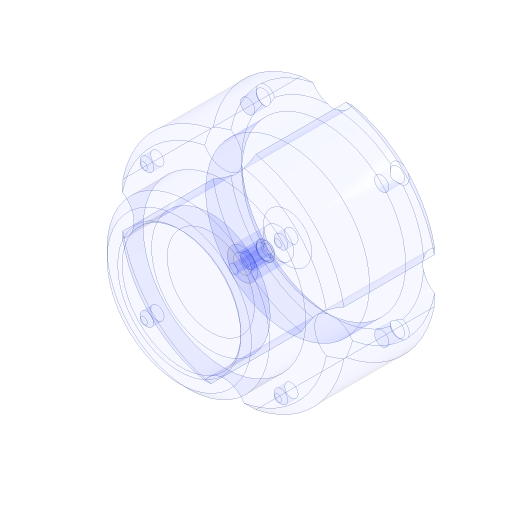
# Autodesk Inventor part: centrifugetool_3.2mm_funnel_v3
Saved by Autodesk Inventor 2024 (Build 280153000, 153)
## iProperties
Created: 2021-10-27
Part Number: centrifugetool_3.2mm_funnel_v3
Material: Generic
Document SubType Name: Modeling
Designer: to172
Density: 1 g/cm^3
Appearance: Clear - Blue
Author: to172
Autodesk Inventor part; units mm, degrees
ref_plane "YZ Plane" through (0, 0, 0) normal (1, 0, 0) x (0, 1, 0)
ref_plane "XZ Plane" through (0, 0, 0) normal (0, 1, 0) x (-1, 0, 0)
ref_plane "XY Plane" through (0, 0, 0) normal (0, 0, 1) x (1, 0, 0)
sketch "Sketch1" plane through (0, 0, 0) normal (0, 0, 1) x (1, 0, 0)
  circle A0 centre (0, 0) radius 12.5
  dimension "d0" = 25
  constraints: 1 centre point, 1 coincident
  measures "d0" diameter of A0
extrude "Extrusion1" add sketch "Sketch1" along normal blind 17
chamfer "Chamfer1" distance 1 angle 45 2 edges at (-12.5, 0, 17) (-12.5, 0, 0)
sketch "Sketch2" plane through (0, 0, 0) normal (0, 1, 0) x (-1, 0, 0)
  line L0 (0, 0) -> (-1.675, 0)
  line L1 (-1.675, 0) -> (-1.675, 10)
  line L2 (0, 17) -> (0, 0)
  line L3 (-0.5, 11) -> (-0.5, 7.2)
  line L4 (-1, 7.2) -> (-1, 10)
  line L5 (-1, 10) -> (-1.675, 10)
  line L6 (-11.5, 17) -> (11.5, 17) projected
  line L7 (0, 17) -> (-5.25, 17)
  line L8 (-1, 7.2) -> (-0.5, 7.2)
  line L9 (-1.675, 0) -> (-9.075, 0)
  line L10 (-9.075, 0) -> (-9.075, 5)
  line L11 (-9.075, 5) -> (-1.675, 5)
  line L12 (-1.675, 5) -> (-1.675, 0)
  line L13 (-1, 9.45) -> (-1.675, 9.45) construction
  line L14 (-0.5, 11) -> (-5.25, 13.7424)
  line L15 (-5.25, 13.7424) -> (-5.25, 17)
  line L16 (12.5, 16) -> (-12.5, 16) projected
  point P0 (-1.675, 5)
  dimension "d7" = 5.25
  dimension "d8" = 1.675
  dimension "d11" = 9.075
  dimension "d12" = 5
  dimension "d13" = 5
  dimension "d14" = 1
  dimension "d15" = 9.45
  dimension "d16" = 2.25
  dimension "d18" = 0.5
  dimension "d41" = 1
  dimension "d42" = 60
  constraints: 31 end point, 4 parallel, 4 perpendicular, 3 point on line, 2 horizontal, 1 collinear, 1 midpoint
  measures "d7" distance from line of L7.end L2
  measures "d8" distance between parallel lines of L1 L2
  measures "d11" distance between parallel lines of L10 L2
  measures "d12" distance between parallel lines of L9 L11
  measures "d13" distance between parallel lines of L5 L11
  measures "d14" distance between parallel lines of L4 L2
  measures "d15" distance between parallel lines of L0 L13
  measures "d16" distance between parallel lines of L13 L8
  measures "d18" distance between parallel lines of L4 L3
  measures "d41" distance from line of L3.start L5
  measures "d42" angle of L2 L14
revolve "Revolution1" cut sketch "Sketch2" angle 360 about axis through (0, 0, 17) along (0, 0, -1)
chamfer "Chamfer2" distance 1 angle 45 2 edges at (-1.675, 0, 5) (-9.075, 0, 0)
chamfer "Chamfer3" distance 0.25 angle 45 1 edges at (-1, 0, 7.2)
sketch "Sketch3" plane through (0, 0, 17) normal (0, 0, 1) x (1, 0, 0)
  circle A0 centre (0, 0) radius 0.5 projected
  circle A1 centre (0, 0) radius 12.5
  circle A2 centre (0, 0) radius 6.575
  circle A3 centre (0, 0) radius 9
  circle A4 centre (0, 0) radius 12.5 projected
  circle A5 centre (-12.5, 0) radius 2.5
  line L0 (0, 0) -> (-12.5, 0) construction
  circle A6 centre (0, -12.5) radius 2.5
  circle A7 centre (12.5, 0) radius 2.5
  circle A8 centre (0, 12.5) radius 2.5
  point P0 (12.25, 2.4875)
  point P1 (12.25, -2.4875)
  point P2 (-2.4875, 12.25)
  point P3 (2.4875, 12.25)
  point P4 (-12.25, 2.4875)
  point P5 (-12.25, -2.4875)
  point P6 (2.4875, -12.25)
  point P7 (-2.4875, -12.25)
  dimension "d27" = 25
  dimension "d28" = 5
  dimension "d31" = 360
  dimension "d33" = 13.15
  dimension "d34" = 18
  constraints: 7 centre point, 3 coincident, 2 end point, 1 horizontal, 1 horizontal alignment, 10 other
  measures "d27" diameter of A1
  measures "d28" diameter of A5
  measures "d33" diameter of A2
  measures "d34" diameter of A3
extrude "Extrusion2" cut sketch "Sketch3" against normal through all contours A1 A7 | A8 A1 | A1 A6 | A5 A1 picked at (11.6823, -0.4803) picked at (0, 11.6481) picked at (0, -11.6481) picked at (-11.6481, 0)
extrude "Extrusion3" cut sketch "Sketch3" against normal blind 5 contours A7 A1 A6 A5 A8
extrude "Extrusion4" cut sketch "Sketch3" against normal blind 3.5 contours A2
chamfer "Chamfer4" distance 0.25 angle 45 1 edges at (-6.575, 0, 17)
chamfer "Chamfer5" distance 1 angle 45 5 edges at (-9, 0, 17) (-8.8388, -8.8388, 12) (8.8388, -8.8388, 12) (8.8388, 8.8388, 12) (-8.8388, 8.8388, 12)
sketch "Sketch4" plane through (0, 0, 12) normal (0, 0, 1) x (1, 0, 0)
  circle A0 centre (0, 0) radius 0.5 construction
  line L0 (0, 0) -> (14.5637, 0) construction
  line L1 (0, 0) -> (0, -17.4879) construction
  circle A1 centre (0, 0) radius 1 construction
  line L2 (0, 0) -> (13.8046, -13.8046) construction
  circle A2 centre (0, 0) radius 10.5 construction
  circle A3 centre (7.4246, -7.4246) radius 0.75
  circle A4 centre (7.4246, 7.4246) radius 0.75
  circle A5 centre (-7.4246, 7.4246) radius 0.75
  circle A6 centre (-7.4246, -7.4246) radius 0.75
  dimension "d50" = 21
  dimension "d49" = 45
  dimension "d51" = 1.5
  dimension "d54" = 360
  constraints: 6 end point, 4 centre point, 1 coincident, 1 horizontal, 1 point on line, 1 vertical, 12 other
  measures "d49" angle of L2 L0
  measures "d51" diameter of A3
extrude "Extrusion5" add sketch "Sketch4" along normal blind 1.5
chamfer "Chamfer6" distance 0.35 angle 45 4 edges at (-8.1746, 7.4246, 13.5) (-8.1746, -7.4246, 13.5) (6.6746, -7.4246, 13.5) (6.6746, 7.4246, 13.5)
sketch "Sketch5" plane through (0, 0, 0) normal (0, 0, -1) x (-1, 0, 0)
  circle A0 centre (0, 0) radius 0 construction
  line L0 (0, 0) -> (14.5637, 0) construction
  line L1 (0, 0) -> (0, -17.4879) construction
  line L2 (0, 0) -> (15.1216, -15.1216) construction
  circle A1 centre (0, 0) radius 10.5 construction
  circle A2 centre (7.4246, -7.4246) radius 0.8
  circle A3 centre (7.4246, 7.4246) radius 0.8
  circle A4 centre (-7.4246, 7.4246) radius 0.8
  circle A5 centre (-7.4246, -7.4246) radius 0.8
  circle A6 centre (0, 0) radius 0.5 projected
  dimension "d64" = 21
  dimension "d63" = 45
  dimension "d65" = 1.6
  dimension "d66" = 360
  constraints: 6 end point, 4 centre point, 2 coincident, 1 horizontal, 1 point on line, 1 vertical, 15 other
  measures "d63" angle of L2 L0
  measures "d65" diameter of A2
extrude "Extrusion6" cut sketch "Sketch5" against normal blind 2 contours A2 | A3 | A4 | A5
chamfer "Chamfer7" distance 0.25 angle 45 6 edges at (-8.0421, -6.916, 0) (-7.5016, -8.2209, 0) (-7.5016, 8.2209, 0) (-8.0421, 6.916, 0) (7.9903, 7.9903, 0) (7.9903, -7.9903, 0)
body "Solid1"
